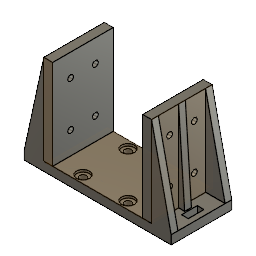
Y Axix Mount for X other Side (Autodesk Fusion 360 design; units mm, degrees)
Autodesk Fusion 360 part; units mm, degrees
sketch "Skizze1" plane through (0, 0, 0) normal (0, 1, 0) x (1, 0, 0)
  line L0 (0, 0) -> (45.4, 0)
  line L1 (0, 0) -> (0, -27)
  line L2 (0, -27) -> (45.4, -27)
  line L3 (45.4, 0) -> (45.4, -27)
  dimension "d1" = 45.4
  dimension "d2" = 27
  dimension "d3" = 45.4
  constraint coincident L0.start L1.start
  constraint horizontal L0
  constraint perpendicular L0 L1
  constraint perpendicular L1 L2
  measures "d1" distance of L0.start L0.end
  measures "d2" distance of L0.start L1.end
  measures "d3" distance of L1.end L2.end
extrude "Extrusion1" add sketch "Skizze1" along normal blind 4
sketch "Skizze2" plane through (0, 4, 0) normal (0, 1, 0) x (-1, 0, 0)
  line L0 (0, 0) -> (0, 27)
  line L1 (0, 27) -> (-45.4, 27)
  line L2 (-45.4, 27) -> (-45.4, 0)
  line L3 (-45.4, 0) -> (0, 0)
  line L4 (0, 0) -> (-12.7, 0)
  circle A0 centre (-12.7, 3.5) radius 1.5
  circle A1 centre (-32.7, 3.5) radius 1.5
  circle A2 centre (-12.7, 23.5) radius 1.5
  circle A3 centre (-32.7, 23.5) radius 1.5
  dimension "d10" = 3
  dimension "d11" = 3
  dimension "d13" = 3
  dimension "d15" = 3
  constraint coincident L0.start L3.end
  constraint perpendicular L0 L4
  measures "d10" diameter of A0
  measures "d11" diameter of A1
  measures "d13" diameter of A2
  measures "d15" diameter of A3
extrude "Extrusion2" cut sketch "Skizze2" against normal blind 41 contours A0 | A1 | A2 | A3
sketch "Skizze3" plane through (0, 4, 0) normal (0, 1, 0) x (-1, 0, 0)
  circle A0 centre (-12.7, 23.5) radius 1.5
  circle A1 centre (-32.7, 23.5) radius 1.5
  circle A2 centre (-12.7, 3.5) radius 1.5
  circle A3 centre (-32.7, 3.5) radius 1.5
  line L0 (0, 0) -> (0, 27)
  line L1 (0, 27) -> (-45.4, 27)
  line L2 (-45.4, 27) -> (-45.4, 0)
  line L3 (-45.4, 0) -> (0, 0)
  circle A4 centre (-12.7, 3.5) radius 2.85
  circle A5 centre (-32.7, 3.5) radius 2.85
  circle A6 centre (-32.7, 23.5) radius 2.85
  circle A7 centre (-12.7, 23.5) radius 2.85
  dimension "d18" = 5.7
  dimension "d19" = 5.7
  dimension "d20" = 5.7
  dimension "d21" = 5.7
  constraint concentric A2 A4
  constraint concentric A3 A5
  constraint concentric A1 A6
  constraint concentric A0 A7
  measures "d18" diameter of A4
  measures "d19" diameter of A5
  measures "d20" diameter of A6
  measures "d21" diameter of A7
extrude "Extrusion3" cut sketch "Skizze3" against normal blind 1 contours A4 | A5 | A6 | A7
sketch "Skizze4" plane through (0, 4, 0) normal (0, 1, 0) x (-1, 0, 0)
  circle A0 centre (-32.7, 3.5) radius 2.85
  circle A1 centre (-32.7, 23.5) radius 2.85
  circle A2 centre (-12.7, 3.5) radius 2.85
  circle A3 centre (-12.7, 23.5) radius 2.85
  line L0 (0, 0) -> (0, 27)
  line L1 (0, 27) -> (-45.4, 27)
  line L2 (-45.4, 27) -> (-45.4, 0)
  line L3 (-45.4, 0) -> (0, 0)
move_face "Flächen versetzen1" offset 10 1 faces at (0, 1.3333, 9)
move_face "Flächen versetzen2" offset 10 1 faces at (45.4, 1.3333, 9)
sketch "Skizze5" plane through (0, 4, 0) normal (0, 1, 0) x (-1, 0, 0)
sketch "Skizze6" plane through (0, 4, 0) normal (0, 1, 0) x (-1, 0, 0)
extrude "Extrusion4" add 1 faces at (-3.2183, 4, 16.2982) along direction (0, 1, 0) blind 2
extrude "Extrusion5" cut 1 faces at (-3.2183, 6, 16.2982) along direction (0, -1, 0) blind 2
sketch "Skizze7" plane through (0, 4, 0) normal (0, 1, 0) x (-1, 0, 0)
  circle A0 centre (-32.7, 3.5) radius 2.85
  circle A1 centre (-32.7, 23.5) radius 2.85
  circle A2 centre (-12.7, 3.5) radius 2.85
  circle A3 centre (-12.7, 23.5) radius 2.85
  line L0 (10, 0) -> (10, 27)
  line L1 (10, 27) -> (-55.4, 27)
  line L2 (-55.4, 27) -> (-55.4, 0)
  line L3 (-55.4, 0) -> (10, 0)
  line L4 (-32.7, 3.5) -> (-42.7, 3.5)
  line L5 (-32.7, 23.5) -> (-42.7, 23.5)
  line L6 (-12.7, 3.5) -> (-2.7, 3.5)
  line L7 (-12.7, 23.5) -> (-2.7, 23.5)
  line L8 (-42.7, 3.5) -> (-42.7, 0)
  line L9 (-42.7, 3.5) -> (-42.7, 27)
  line L10 (-2.7, 23.5) -> (-2.7, -1)
  line L11 (-2.7, -1) -> (-2.7, 27)
  line L12 (-42.7, 0) -> (-46.7, 0)
  line L13 (-46.7, 0) -> (-46.7, 27)
  line L14 (-42.7, 27) -> (-46.7, 27)
  line L15 (-2.7, 3.5) -> (-2.7, 0)
  line L16 (-2.7, 0) -> (1.3, 0)
  line L17 (1.3, 0) -> (1.3, 27)
  line L18 (1.3, 27) -> (-2.7, 27)
  dimension "d34" = 10
  dimension "d35" = 10
  dimension "d36" = 10
  dimension "d37" = 10
  dimension "d38" = 4
  dimension "d39" = 4
  constraint coincident A0.centre L4.start
  constraint parallel L3 L4
  constraint coincident A1.centre L5.start
  constraint parallel L3 L5
  constraint coincident A2.centre L6.start
  constraint parallel L3 L6
  constraint coincident A3.centre L7.start
  constraint horizontal L7
  constraint coincident L3 L8.end
  constraint perpendicular L4 L8
  constraint coincident L1 L9.end
  constraint perpendicular L1 L9
  constraint perpendicular L3 L10
  constraint coincident L1 L11.end
  constraint perpendicular L1 L11
  constraint perpendicular L8 L12
  constraint coincident L1 L13.end
  constraint perpendicular L1 L13
  constraint coincident L3 L15.end
  constraint coincident L10 L15.end
  constraint perpendicular L11 L16
  constraint coincident L1 L17.end
  constraint perpendicular L1 L17
  measures "d34" distance of A0.centre L4.end
  measures "d35" distance of A1.centre L5.end
  measures "d36" distance of A2.centre L6.end
  measures "d37" distance of A3.centre L7.end
  measures "d38" distance of L8.end L12.end
  measures "d39" distance of L15.end L16.end
extrude "Extrusion6" add sketch "Skizze7" along normal blind 40 contours L1 L3 L10 L11 L15 L16 L17 L18 | L1 L3 L8 L9 L12 L13 L14
sketch "Skizze8" plane through (0, 4, 0) normal (0, 1, 0) x (-1, 0, 0)
sketch "Skizze9" plane through (46.7, 0, 0) normal (1, 0, 0) x (0, 0, -1)
  line L0 (-27, 4) -> (0, 4)
  line L1 (0, 4) -> (0, 44)
  line L2 (0, 44) -> (-27, 44)
  line L3 (-27, 44) -> (-27, 4)
sketch "Skizze10" plane through (46.7, 0, 0) normal (1, 0, 0) x (0, 1, 0)
  line L0 (44, 27) -> (44, 19)
  line L1 (44, 0) -> (44, 8)
  circle A0 centre (34, 19) radius 1.275
  circle A1 centre (34, 8) radius 1.275
  circle A2 centre (14, 19) radius 1.275
  circle A3 centre (14, 8) radius 1.275
  dimension "d46" = 2.55
  dimension "d47" = 2.55
  dimension "d50" = 2.55
  dimension "d51" = 2.55
  constraint vertical L0
  constraint vertical L1
  measures "d46" diameter of A0
  measures "d47" diameter of A1
  measures "d50" diameter of A2
  measures "d51" diameter of A3
extrude "Extrusion7" cut sketch "Skizze10" against normal blind 71
sketch "Skizze11" plane through (46.7, 0, 0) normal (1, 0, 0) x (0, 0, -1)
  line L0 (-27, 44) -> (-24, 44)
  line L1 (-24, 44) -> (-24, 4)
  line L2 (-27, 4) -> (-24, 4)
  line L3 (-27, 4) -> (-27, 44)
  line L4 (0, 44) -> (-3, 44)
  line L5 (-3, 44) -> (-3, 4)
  line L6 (-3, 4) -> (0, 4)
  line L7 (0, 4) -> (0, 44)
  constraint horizontal L0
  constraint perpendicular L0 L1
  constraint perpendicular L1 L2
  constraint perpendicular L0 L3
  constraint perpendicular L1 L4
  constraint perpendicular L4 L5
  constraint perpendicular L5 L6
  constraint perpendicular L4 L7
extrude "Extrusion8" add sketch "Skizze11" along normal blind 8.7
sketch "Skizze12" plane through (0, 0, 27) normal (0, 0, 1) x (1, 0, 0)
  line L0 (46.7, 4) -> (42.7, 4)
  line L1 (42.7, 4) -> (2.7, 4)
  line L2 (2.7, 4) -> (-1.3, 4)
  line L3 (-1.3, 4) -> (-10, 4)
  line L4 (-10, 4) -> (-10, 0)
  line L5 (-10, 0) -> (55.4, 0)
  line L6 (55.4, 0) -> (55.4, 44)
  line L7 (55.4, 44) -> (46.7, 44)
  line L8 (46.7, 44) -> (46.7, 4)
  line L9 (46.7, 44) -> (55.4, 4)
  constraint coincident L7.end L8.start
  constraint coincident L6 L9.end
extrude "Extrusion9" cut sketch "Skizze12" against normal blind 41 contours L6 L7 L9
sketch "Skizze13" plane through (-1.3, 0, 0) normal (-1, 0, 0) x (0, 0, 1)
  circle A0 centre (19, 34) radius 1.275
  circle A1 centre (19, 14) radius 1.275
  circle A2 centre (8, 34) radius 1.275
  circle A3 centre (8, 14) radius 1.275
  line L0 (0, 4) -> (27, 4)
  line L1 (27, 4) -> (27, 44)
  line L2 (27, 44) -> (0, 44)
  line L3 (0, 44) -> (0, 4)
  line L4 (0, 44) -> (3, 44)
  line L5 (3, 44) -> (3, 4)
  line L6 (3, 4) -> (0, 4)
  line L7 (0, 4) -> (0, 44)
  line L8 (27, 44) -> (24, 44)
  line L9 (24, 44) -> (24, 43.5002)
  line L10 (24, 43.5002) -> (24, 4)
  line L11 (24, 4) -> (27, 4)
  line L12 (27, 4) -> (27, 44)
  constraint coincident L2.end L3.start
  constraint coincident L2 L4.end
  constraint perpendicular L3 L4
  constraint coincident L0 L5.end
  constraint perpendicular L0 L5
  constraint coincident L0.start L3.end
  constraint coincident L1.end L2.start
  constraint coincident L2 L8.end
  constraint perpendicular L1 L8
  constraint perpendicular L2 L9
  constraint coincident L0 L10.end
  constraint perpendicular L0 L10
  constraint coincident L0.end L1.start
extrude "Extrusion10" add sketch "Skizze13" along normal blind 8.7 contours L0 L2 L3 L4 L5 L6 L7 | L0 L1 L2 L8 L9 L10 L11 L12
sketch "Skizze14" plane through (0, 0, 27) normal (0, 0, 1) x (1, 0, 0)
  line L0 (55.4, 4) -> (46.7, 44)
  line L1 (46.7, 44) -> (46.7, 4)
  line L2 (46.7, 4) -> (42.7, 4)
  line L3 (42.7, 4) -> (2.7, 4)
  line L4 (2.7, 4) -> (-1.3, 4)
  line L5 (-1.3, 4) -> (-1.3, 44)
  line L6 (-1.3, 44) -> (-10, 44)
  line L7 (-10, 44) -> (-10, 0)
  line L8 (-10, 0) -> (55.4, 0)
  line L9 (55.4, 0) -> (55.4, 4)
  line L10 (-1.3, 44) -> (-10, 3.9822)
  constraint coincident L5.end L6.start
  constraint coincident L7 L10.end
extrude "Extrusion11" cut sketch "Skizze14" against normal blind 38 contours L6 L7 L10
sketch "Skizze15" plane through (46.7, 0, 0) normal (1, 0, 0) x (0, 0, -1)
  line L0 (-19, 34) -> (-13.5, 34)
  line L1 (-13.5, 34) -> (-13.5, 44)
  line L2 (-13.5, 44) -> (-15, 44)
  line L3 (-15, 44) -> (-15, 4)
  line L4 (-13.5, 44) -> (-12, 44)
  line L5 (-12, 44) -> (-12, 4)
  line L6 (-15, 4) -> (-12, 4)
  dimension "d62" = 5.5
  dimension "d63" = 40
  dimension "d64" = 40
  constraint horizontal L0
  constraint perpendicular L0 L1
  constraint perpendicular L1 L2
  constraint perpendicular L0 L3
  constraint perpendicular L1 L4
  constraint perpendicular L2 L5
  measures "d62" distance of L0.start L0.end
  measures "d63" distance of L2.end L3.end
  measures "d64" distance of L4.end L5.end
extrude "Extrusion12" add sketch "Skizze15" along normal blind 2.7
sketch "Skizze16" plane through (0, 4, 0) normal (0, 1, 0) x (-1, 0, 0)
  line L0 (-49.4, 15) -> (-46.7, 15)
  line L1 (-46.7, 15) -> (-46.7, 24)
  line L2 (-46.7, 24) -> (-55.4, 24)
  line L3 (-55.4, 24) -> (-55.4, 3)
  line L4 (-55.4, 3) -> (-46.7, 3)
  line L5 (-46.7, 3) -> (-46.7, 12)
  line L6 (-46.7, 12) -> (-49.4, 12)
  line L7 (-49.4, 12) -> (-49.4, 15)
  line L8 (-50, 12) -> (-50, 15)
  line L9 (-50, 15) -> (-50, 17)
  line L10 (-50, 17) -> (-50, 12)
  line L11 (-50, 12) -> (-50, 10)
  line L12 (-50, 10) -> (-53, 10)
  line L13 (-53, 10) -> (-53, 17)
  line L14 (-53, 17) -> (-50, 17)
  constraint perpendicular L6 L8
  constraint perpendicular L6 L9
  constraint parallel L8 L11
  constraint perpendicular L11 L12
  constraint perpendicular L12 L13
  constraint perpendicular L9 L14
extrude "Extrusion13" cut sketch "Skizze16" against normal blind 13 contours L8 L9 L10 L11 L12 L13 L14
sketch "Skizze17" plane through (0, 0, 15) normal (0, 0, 1) x (1, 0, 0)
  line L0 (46.7, 44) -> (46.7, 4)
  line L1 (46.7, 4) -> (49.4, 4)
  line L2 (49.4, 4) -> (49.4, 44)
  line L3 (49.4, 44) -> (46.7, 44)
  line L4 (46.7, 44) -> (49.4, 4)
  constraint coincident L0.start L3.end
  constraint coincident L1.end L2.start
extrude "Extrusion14" cut sketch "Skizze17" against normal blind 3 contours L2 L3 L4
sketch "Skizze18" plane through (-1.3, 0, 0) normal (-1, 0, 0) x (0, 0, 1)
  circle A0 centre (8, 14) radius 1.275
  circle A1 centre (8, 34) radius 1.275
  circle A2 centre (19, 14) radius 1.275
  circle A3 centre (19, 34) radius 1.275
  line L0 (3, 44) -> (3, 4)
  line L1 (3, 4) -> (24, 4)
  line L2 (24, 4) -> (24, 44)
  line L3 (24, 44) -> (3, 44)
  line L4 (8, 34) -> (13.5, 34)
  line L5 (13.5, 34) -> (13.5, 44)
  line L6 (13.5, 44) -> (12, 44)
  line L7 (12, 44) -> (12, 4)
  line L8 (13.5, 44) -> (15, 44)
  line L9 (15, 44) -> (15, 4)
  line L10 (12, 4) -> (15, 4)
  dimension "d71" = 5.5
  dimension "d72" = 40
  dimension "d73" = 40
  constraint coincident A1.centre L4.start
  constraint perpendicular L0 L4
  constraint midpoint L3 L5.end
  constraint coincident L3 L6.end
  constraint parallel L3 L6
  constraint perpendicular L3 L7
  constraint coincident L3 L8.end
  constraint parallel L3 L8
  constraint perpendicular L8 L9
  measures "d71" distance of A1.centre L4.end
  measures "d72" distance of L6.end L7.end
  measures "d73" distance of L8.end L9.end
extrude "Extrusion15" add sketch "Skizze18" along normal blind 2.7 contours L3 L4 L5 L6 L7 | L1 L3 L4 L5 L7 L8 L9 L10
sketch "Skizze19" plane through (0, 4, 0) normal (0, 1, 0) x (-1, 0, 0)
  line L0 (4, 12) -> (1.3, 12)
  line L1 (1.3, 12) -> (1.3, 3)
  line L2 (1.3, 3) -> (9.9961, 3)
  line L3 (9.9961, 3) -> (9.9961, 24)
  line L4 (9.9961, 24) -> (1.3, 24)
  line L5 (1.3, 24) -> (1.3, 15)
  line L6 (1.3, 15) -> (4, 15)
  line L7 (4, 15) -> (4, 12)
  line L8 (4, 12) -> (4.6, 12)
  line L9 (4.6, 12) -> (4.6, 15)
  line L10 (4.6, 15) -> (4.6, 17)
  line L11 (4.6, 17) -> (7.6, 17)
  line L12 (4.6, 12) -> (4.6, 10)
  line L13 (4.6, 10) -> (7.6, 10)
  line L14 (7.6, 10) -> (7.6, 17)
  dimension "d76" = 0.6
  dimension "d77" = 3
  dimension "d78" = 2
  dimension "d79" = 3
  constraint coincident L0.start L7.end
  constraint perpendicular L7 L8
  constraint perpendicular L8 L9
  constraint perpendicular L8 L10
  constraint perpendicular L10 L11
  constraint perpendicular L8 L12
  constraint perpendicular L12 L13
  measures "d76" distance of L0.start L8.end
  measures "d77" distance of L10.end L11.end
  measures "d78" distance of L8.end L12.end
  measures "d79" distance of L12.end L13.end
extrude "Extrusion16" cut sketch "Skizze19" against normal blind 15 contours L9 L10 L11 L12 L13 L14
sketch "Skizze20" plane through (0, 0, 15) normal (0, 0, 1) x (1, 0, 0)
  line L0 (-1.3, 4) -> (-1.3, 44)
  line L1 (-1.3, 44) -> (-4, 44)
  line L2 (-4, 44) -> (-4, 4)
  line L3 (-4, 4) -> (-1.3, 4)
  line L4 (-1.3, 44) -> (-4, 4)
  constraint coincident L0.end L1.start
  constraint coincident L2.end L3.start
extrude "Extrusion17" cut sketch "Skizze20" against normal blind 3 contours L1 L2 L4
sketch "Skizze21" plane through (0, 0, 27) normal (0, 0, 1) x (1, 0, 0)
  line L0 (-1.3, 4) -> (2.7, 4)
  line L1 (2.7, 4) -> (2.7, 44)
  line L2 (2.7, 44) -> (-1.3, 44)
  line L3 (-1.3, 44) -> (-1.3, 4)
